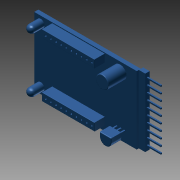
# Autodesk Inventor part: Adafruit xbee adapter
Saved by Autodesk Inventor 2012 (Build 160160000, 160)
## iProperties
Created: 2012-03-02
Part Number: Adafruit xbee adapter
Material: Default
Document SubType Name: Modeling
Designer: Lauszus
Density: 1 g/cm^3
Author: Lauszus
Autodesk Inventor part; units mm, degrees
ref_plane "YZ Plane" through (0, 0, 0) normal (1, 0, 0) x (0, 1, 0)
ref_plane "XZ Plane" through (0, 0, 0) normal (0, 1, 0) x (-1, 0, 0)
ref_plane "XY Plane" through (0, 0, 0) normal (0, 0, 1) x (1, 0, 0)
sketch "Sketch1" plane through (0, 0, 0) normal (0, 0, 1) x (1, 0, 0)
  line L0 (22.2522, -7.5943) -> (-17.7478, -7.5943)
  line L1 (-17.7478, -7.5943) -> (-17.7478, 18.9057)
  line L2 (-17.7478, 18.9057) -> (22.2522, 18.9057)
  line L3 (22.2522, 18.9057) -> (22.2522, -7.5943)
  line L4 (-10.7478, 18.5791) -> (9.7522, 18.5791)
  line L5 (9.7522, 18.5791) -> (9.7522, 15.5791)
  line L6 (9.7522, 15.5791) -> (-10.7478, 15.5791)
  line L7 (-10.7478, 15.5791) -> (-10.7478, 18.5791)
  circle A0 centre (-15.2478, -5.0275) radius 1.5
  circle A1 centre (-15.2478, 16.3389) radius 1.5
  circle A2 centre (15.7522, 15.4057) radius 2.5
  line L8 (18.2522, -4.3443) -> (18.2522, -2.8443)
  line L9 (18.2522, -2.8443) -> (13.7522, -2.8443)
  line L10 (13.7522, -2.8443) -> (13.7522, -4.3443)
  arc A3 (13.7522, -4.3443) -> (18.2522, -4.3443) centre (16.0022, -4.3443) ccw
  line L11 (14.295, -3.3443) -> (14.795, -3.3443)
  line L12 (14.795, -3.3443) -> (14.795, -3.8443)
  line L13 (14.795, -3.8443) -> (14.295, -3.8443)
  line L14 (14.295, -3.8443) -> (14.295, -3.3443)
  line L15 (15.795, -3.3443) -> (16.295, -3.3443)
  line L16 (16.295, -3.3443) -> (16.295, -3.8443)
  line L17 (16.295, -3.8443) -> (15.795, -3.8443)
  line L18 (15.795, -3.8443) -> (15.795, -3.3443)
  line L19 (17.295, -3.3443) -> (17.795, -3.3443)
  line L20 (17.795, -3.3443) -> (17.795, -3.8443)
  line L21 (17.795, -3.8443) -> (17.295, -3.8443)
  line L22 (17.295, -3.8443) -> (17.295, -3.3443)
  line L23 (-9.6556, 17.3791) -> (-9.0556, 17.3791)
  line L24 (-9.0556, 17.3791) -> (-9.0556, 16.7791)
  line L25 (-9.0556, 16.7791) -> (-9.6556, 16.7791)
  line L26 (-9.6556, 16.7791) -> (-9.6556, 17.3791)
  line L27 (-7.6556, 17.3791) -> (-7.0556, 17.3791)
  line L28 (-7.0556, 17.3791) -> (-7.0556, 16.7791)
  line L29 (-7.0556, 16.7791) -> (-7.6556, 16.7791)
  line L30 (-7.6556, 16.7791) -> (-7.6556, 17.3791)
  line L31 (-5.6556, 16.7791) -> (-5.0556, 16.7791)
  line L32 (-5.0556, 16.7791) -> (-5.0556, 17.3791)
  line L33 (-5.0556, 17.3791) -> (-5.6556, 17.3791)
  line L34 (-5.6556, 17.3791) -> (-5.6556, 16.7791)
  line L35 (-3.6556, 16.7791) -> (-3.0556, 16.7791)
  line L36 (-3.0556, 16.7791) -> (-3.0556, 17.3791)
  line L37 (-3.0556, 17.3791) -> (-3.6556, 17.3791)
  line L38 (-3.6556, 17.3791) -> (-3.6556, 16.7791)
  line L39 (-1.6556, 16.7791) -> (-1.0556, 16.7791)
  line L40 (-1.0556, 16.7791) -> (-1.0556, 17.3791)
  line L41 (-1.0556, 17.3791) -> (-1.6556, 17.3791)
  line L42 (-1.6556, 17.3791) -> (-1.6556, 16.7791)
  line L43 (0.3444, 16.7791) -> (0.9444, 16.7791)
  line L44 (0.9444, 16.7791) -> (0.9444, 17.3791)
  line L45 (0.9444, 17.3791) -> (0.3444, 17.3791)
  line L46 (0.3444, 17.3791) -> (0.3444, 16.7791)
  line L47 (2.3444, 16.7791) -> (2.9444, 16.7791)
  line L48 (2.9444, 16.7791) -> (2.9444, 17.3791)
  line L49 (2.9444, 17.3791) -> (2.3444, 17.3791)
  line L50 (2.3444, 17.3791) -> (2.3444, 16.7791)
  line L51 (4.3444, 16.7791) -> (4.9444, 16.7791)
  line L52 (4.9444, 16.7791) -> (4.9444, 17.3791)
  line L53 (4.9444, 17.3791) -> (4.3444, 17.3791)
  line L54 (4.3444, 17.3791) -> (4.3444, 16.7791)
  line L55 (6.3444, 16.7791) -> (6.9444, 16.7791)
  line L56 (6.9444, 16.7791) -> (6.9444, 17.3791)
  line L57 (6.9444, 17.3791) -> (6.3444, 17.3791)
  line L58 (6.3444, 17.3791) -> (6.3444, 16.7791)
  line L59 (8.3444, 16.7791) -> (8.9444, 16.7791)
  line L60 (8.9444, 16.7791) -> (8.9444, 17.3791)
  line L61 (8.9444, 17.3791) -> (8.3444, 17.3791)
  line L62 (8.3444, 17.3791) -> (8.3444, 16.7791)
  line L63 (-10.7478, -2.7689) -> (9.7522, -2.7689)
  line L64 (9.7522, -2.7689) -> (9.7522, -5.7689)
  line L65 (9.7522, -5.7689) -> (-10.7478, -5.7689)
  line L66 (-10.7478, -5.7689) -> (-10.7478, -2.7689)
  line L67 (-9.6556, -3.9689) -> (-9.0556, -3.9689)
  line L68 (-9.0556, -3.9689) -> (-9.0556, -4.5689)
  line L69 (-9.0556, -4.5689) -> (-9.6556, -4.5689)
  line L70 (-9.6556, -4.5689) -> (-9.6556, -3.9689)
  line L71 (-7.6556, -3.9689) -> (-7.0556, -3.9689)
  line L72 (-7.0556, -3.9689) -> (-7.0556, -4.5689)
  line L73 (-7.0556, -4.5689) -> (-7.6556, -4.5689)
  line L74 (-7.6556, -4.5689) -> (-7.6556, -3.9689)
  line L75 (-5.6556, -4.5689) -> (-5.0556, -4.5689)
  line L76 (-5.0556, -4.5689) -> (-5.0556, -3.9689)
  line L77 (-5.0556, -3.9689) -> (-5.6556, -3.9689)
  line L78 (-5.6556, -3.9689) -> (-5.6556, -4.5689)
  line L79 (-3.6556, -4.5689) -> (-3.0556, -4.5689)
  line L80 (-3.0556, -4.5689) -> (-3.0556, -3.9689)
  line L81 (-3.0556, -3.9689) -> (-3.6556, -3.9689)
  line L82 (-3.6556, -3.9689) -> (-3.6556, -4.5689)
  line L83 (-1.6556, -4.5689) -> (-1.0556, -4.5689)
  line L84 (-1.0556, -4.5689) -> (-1.0556, -3.9689)
  line L85 (-1.0556, -3.9689) -> (-1.6556, -3.9689)
  line L86 (-1.6556, -3.9689) -> (-1.6556, -4.5689)
  line L87 (0.3444, -4.5689) -> (0.9444, -4.5689)
  line L88 (0.9444, -4.5689) -> (0.9444, -3.9689)
  line L89 (0.9444, -3.9689) -> (0.3444, -3.9689)
  line L90 (0.3444, -3.9689) -> (0.3444, -4.5689)
  line L91 (2.3444, -4.5689) -> (2.9444, -4.5689)
  line L92 (2.9444, -4.5689) -> (2.9444, -3.9689)
  line L93 (2.9444, -3.9689) -> (2.3444, -3.9689)
  line L94 (2.3444, -3.9689) -> (2.3444, -4.5689)
  line L95 (4.3444, -4.5689) -> (4.9444, -4.5689)
  line L96 (4.9444, -4.5689) -> (4.9444, -3.9689)
  line L97 (4.9444, -3.9689) -> (4.3444, -3.9689)
  line L98 (4.3444, -3.9689) -> (4.3444, -4.5689)
  line L99 (6.3444, -4.5689) -> (6.9444, -4.5689)
  line L100 (6.9444, -4.5689) -> (6.9444, -3.9689)
  line L101 (6.9444, -3.9689) -> (6.3444, -3.9689)
  line L102 (6.3444, -3.9689) -> (6.3444, -4.5689)
  line L103 (8.3444, -4.5689) -> (8.9444, -4.5689)
  line L104 (8.9444, -4.5689) -> (8.9444, -3.9689)
  line L105 (8.9444, -3.9689) -> (8.3444, -3.9689)
  line L106 (8.3444, -3.9689) -> (8.3444, -4.5689)
  dimension "d0" = 40
  dimension "d1" = 26.5
  dimension "d3" = 20.5
  dimension "d4" = 3
  dimension "d6" = 7
  dimension "d8" = 3
  dimension "d9" = 3
  dimension "d10" = 1
  dimension "d11" = 1
  dimension "d12" = 5
  dimension "d13" = 4
  dimension "d14" = 1
  dimension "d23" = 1.5
  dimension "d24" = 4.5
  dimension "d28" = 1
  dimension "d29" = 4
  dimension "d33" = 0.5
  dimension "d34" = 0.5
  dimension "d35" = 0.5
  dimension "d36" = 0.5
  dimension "d37" = 0.5
  dimension "d38" = 0.5
  dimension "d39" = 1
  dimension "d40" = 1
  dimension "d41" = 0.5
  dimension "d42" = 0.5
  dimension "d43" = 0.5
  dimension "d44" = 0.4572
  dimension "d56" = 1.0668
  dimension "d58" = 1.0668
  dimension "d191" = 0.6
  dimension "d192" = 0.6
  dimension "d193" = 1.0922
  dimension "d194" = 1.2
  dimension "d195" = 0.6
  dimension "d196" = 0.6
  dimension "d197" = 2
  dimension "d198" = 1.2
  dimension "d199" = 0.6
  dimension "d200" = 0.6
  dimension "d202" = 1.2
  dimension "d203" = 0.6
  dimension "d204" = 0.6
  dimension "d205" = 2
  dimension "d206" = 2
  dimension "d207" = 2
  dimension "d208" = 0.6
  dimension "d209" = 0.6
  dimension "d210" = 1.2
  dimension "d211" = 0.6
  dimension "d212" = 0.6
  dimension "d213" = 2
  dimension "d214" = 1.2
  dimension "d215" = 0.6
  dimension "d216" = 0.6
  dimension "d217" = 2
  dimension "d218" = 1.2
  dimension "d219" = 0.6
  dimension "d220" = 0.6
  dimension "d221" = 2
  dimension "d222" = 1.2
  dimension "d223" = 0.6
  dimension "d224" = 0.6
  dimension "d225" = 2
  constraints: 214 end point, 53 parallel, 26 horizontal, 26 perpendicular, 4 centre point, 2 point on circle, 2 point on line, 2 tangent
  measures "d0" distance of L1.end L2.end
  measures "d1" distance of L0.end L1.end
  measures "d3" distance of L4.start L4.end
  measures "d4" distance of L6.end L4.start
  measures "d6" distance between parallel lines of L1 L7
  measures "d8" diameter of A1
  measures "d9" diameter of A0
  measures "d10" distance edge to line of A0 L1
  measures "d11" distance edge to line of A1 L1
  measures "d12" diameter of A2
  measures "d13" distance edge to line of A2 L3
  measures "d14" distance edge to line of A2 L2
  measures "d23" distance of L8.start L8.end
  measures "d24" distance of L8.end L9.end
  measures "d28" distance edge to line of A3 L0
  measures "d29" distance between parallel lines of L3 L8
  measures "d33" distance of L19.start L19.end
  measures "d34" distance of L19.end L20.end
  measures "d35" distance of L15.end L16.end
  measures "d36" distance of L16.end L17.end
  measures "d37" distance of L11.end L12.end
  measures "d38" distance of L12.end L13.end
  measures "d39" distance between parallel lines of L16 L22
  measures "d40" distance between parallel lines of L12 L18
  measures "d41" distance between parallel lines of L9 L19
  measures "d42" distance between parallel lines of L9 L15
  measures "d43" distance between parallel lines of L9 L11
  measures "d44" distance between parallel lines of L8 L20
  measures "d56" distance edge to line of A1 L2
  measures "d58" distance edge to line of A0 L0
  measures "d191" distance of L23.start L23.end
  measures "d192" distance of L23.end L24.end
  measures "d193" distance between parallel lines of L7 L26
  measures "d194" distance between parallel lines of L6 L25
  measures "d195" distance of L27.start L27.end
  measures "d196" distance of L27.end L28.end
  measures "d197" distance between parallel lines of L26 L30
  measures "d198" distance between parallel lines of L6 L29
  measures "d199" distance of L32.end L33.end
  measures "d200" distance of L33.end L31.start
  measures "d202" distance between parallel lines of L6 L31
  measures "d203" distance of L37.end L35.start
  measures "d204" distance of L36.end L37.end
  measures "d205" distance between parallel lines of L34 L38
  measures "d206" distance between parallel lines of L30 L34
  measures "d207" distance between parallel lines of L38 L42
  measures "d208" distance of L40.end L41.end
  measures "d209" distance of L39.end L40.end
  measures "d210" distance between parallel lines of L6 L39
  measures "d211" distance of L44.end L45.end
  measures "d212" distance of L43.end L44.end
  measures "d213" distance between parallel lines of L42 L46
  measures "d214" distance between parallel lines of L6 L43
  measures "d215" distance of L48.end L49.end
  measures "d216" distance of L47.end L48.end
  measures "d217" distance between parallel lines of L46 L50
  measures "d218" distance between parallel lines of L6 L47
  measures "d219" distance of L52.end L53.end
  measures "d220" distance of L51.end L52.end
  measures "d221" distance between parallel lines of L50 L54
  measures "d222" distance between parallel lines of L6 L51
  measures "d223" distance of L56.end L57.end
  measures "d224" distance of L55.end L56.end
  measures "d225" distance between parallel lines of L54 L58
extrude "Extrusion1" add sketch "Sketch1" against normal blind 1.6 contours L0 L1 L2 L3 | L4 L5 L6 L7 | A0 | A1 | A2 | A3 L10 L9 L8 | L11 L12 L13 L14 | L15 L16 L17 L18 | L19 L20 L21 L22 | L23 L24 L25 L26 | L27 L28 L29 L30 | L34 L33 L32 L31 | L38 L37 L36 L35 | L42 L41 L40 L39 | L46 L45 L44 L43 | L50 L49 L48 L47 | L54 L53 L52 L51 | L58 L57 L56 L55 | L62 L61 L60 L59 | L63 L64 L65 L66 | L67 L68 L69 L70 | L71 L72 L73 L74 | L78 L77 L76 L75 | L82 L81 L80 L79 | L86 L85 L84 L83 | L90 L89 L88 L87 | L94 L93 L92 L91 | L98 L97 L96 L95 | L102 L101 L100 L99 | L106 L105 L104 L103
extrude "Extrusion2" add sketch "Sketch1" along normal blind 7 contours A2
extrude "Extrusion3" add sketch "Sketch1" along normal blind 5 contours A0 | A1
fillet "Fillet1" radius 1.4986 2 edges at (-16.7478, -5.0275, 5) (-16.7478, 16.3389, 5)
fillet "Fillet2" radius 0.254 1 edges at (13.2522, 15.4057, 7)
extrude "Extrusion5" add sketch "Sketch1" along normal blind 2 contours L11 L12 L13 L14 | L15 L16 L17 L18 | L19 L20 L21 L22
sketch "Sketch3" plane through (22.2522, -7.5943, 0) normal (1, 0, 0) x (0, 0, -1)
  line L0 (0, 0) -> (1.6, 0) projected
  line L1 (0.8, 0) -> (2.5, 0)
  line L2 (2.5, 0) -> (2.5, 26.5)
  line L3 (2.5, 26.5) -> (0.8, 26.5)
  line L4 (0.8, 26.5) -> (0.8, 0)
  line L5 (1.9, 2.0621) -> (1.4, 2.0621)
  line L6 (1.4, 2.0621) -> (1.4, 1.5621)
  line L7 (1.4, 1.5621) -> (1.9, 1.5621)
  line L8 (1.9, 1.5621) -> (1.9, 2.0621)
  line L9 (1.9, 4.1021) -> (1.4, 4.1021)
  line L10 (1.4, 4.1021) -> (1.4, 4.6021)
  line L11 (1.4, 4.6021) -> (1.9, 4.6021)
  line L12 (1.9, 4.6021) -> (1.9, 4.1021)
  line L13 (1.9, 6.6421) -> (1.4, 6.6421)
  line L14 (1.4, 6.6421) -> (1.4, 7.1421)
  line L15 (1.4, 7.1421) -> (1.9, 7.1421)
  line L16 (1.9, 7.1421) -> (1.9, 6.6421)
  line L17 (1.9, 9.6821) -> (1.4, 9.6821)
  line L18 (1.4, 9.6821) -> (1.4, 9.1821)
  line L19 (1.4, 9.1821) -> (1.9, 9.1821)
  line L20 (1.9, 9.1821) -> (1.9, 9.6821)
  line L21 (1.9, 12.2221) -> (1.4, 12.2221)
  line L22 (1.4, 12.2221) -> (1.4, 11.7221)
  line L23 (1.4, 11.7221) -> (1.9, 11.7221)
  line L24 (1.9, 11.7221) -> (1.9, 12.2221)
  line L25 (1.9, 14.7621) -> (1.4, 14.7621)
  line L26 (1.4, 14.7621) -> (1.4, 14.2621)
  line L27 (1.4, 14.2621) -> (1.9, 14.2621)
  line L28 (1.9, 14.2621) -> (1.9, 14.7621)
  line L29 (1.9, 17.3021) -> (1.4, 17.3021)
  line L30 (1.4, 17.3021) -> (1.4, 16.8021)
  line L31 (1.4, 16.8021) -> (1.9, 16.8021)
  line L32 (1.9, 16.8021) -> (1.9, 17.3021)
  line L33 (1.4, 19.3421) -> (1.9, 19.3421)
  line L34 (1.9, 19.3421) -> (1.9, 19.8421)
  line L35 (1.9, 19.8421) -> (1.4, 19.8421)
  line L36 (1.4, 19.8421) -> (1.4, 19.3421)
  line L37 (1.4, 21.8821) -> (1.9, 21.8821)
  line L38 (1.9, 21.8821) -> (1.9, 22.3821)
  line L39 (1.9, 22.3821) -> (1.4, 22.3821)
  line L40 (1.4, 22.3821) -> (1.4, 21.8821)
  line L41 (1.4, 24.4221) -> (1.9, 24.4221)
  line L42 (1.9, 24.4221) -> (1.9, 24.9221)
  line L43 (1.9, 24.9221) -> (1.4, 24.9221)
  line L44 (1.4, 24.9221) -> (1.4, 24.4221)
  point P0 (0, 7.5943)
  dimension "d122" = 26.5
  dimension "d123" = 1.7
  dimension "d124" = 0.5
  dimension "d125" = 0.5
  dimension "d126" = 1.5621
  dimension "d127" = 0.6
  dimension "d128" = 0.5
  dimension "d129" = 0.5
  dimension "d130" = 0.5
  dimension "d131" = 0.5
  dimension "d145" = 0.6
  dimension "d147" = 0.6
  dimension "d148" = 0.5
  dimension "d149" = 0.5
  dimension "d150" = 2.54
  dimension "d151" = 0.6
  dimension "d152" = 2.54
  dimension "d154" = 0.5
  dimension "d155" = 0.5
  dimension "d156" = 2.54
  dimension "d157" = 0.6
  dimension "d158" = 0.5
  dimension "d159" = 0.5
  dimension "d160" = 2.54
  dimension "d161" = 0.6
  dimension "d162" = 2.54
  dimension "d163" = 0.5
  dimension "d164" = 0.5
  dimension "d166" = 2.54
  dimension "d167" = 0.6
  dimension "d168" = 0.5
  dimension "d169" = 0.5
  dimension "d170" = 2.54
  dimension "d171" = 0.6
  dimension "d172" = 0.5
  dimension "d173" = 0.5
  dimension "d174" = 2.54
  dimension "d175" = 0.6
  dimension "d176" = 0.5
  dimension "d177" = 0.5
  dimension "d178" = 2.54
  dimension "d179" = 0.6
  constraints: 88 end point, 22 parallel, 11 horizontal, 11 perpendicular, 1 midpoint
  measures "d122" distance of L1.end L2.end
  measures "d123" distance of L2.end L3.end
  measures "d124" distance of L5.end L6.end
  measures "d125" distance of L5.start L5.end
  measures "d126" distance from line of L1 L6.end
  measures "d127" distance between parallel lines of L4 L6
  measures "d128" distance of L10.end L11.end
  measures "d129" distance of L9.end L10.end
  measures "d130" distance of L15.start L15.end
  measures "d131" distance of L14.start L15.start
  measures "d145" distance between parallel lines of L4 L10
  measures "d147" distance between parallel lines of L4 L14
  measures "d148" distance of L17.end L18.end
  measures "d149" distance of L17.start L17.end
  measures "d150" distance from line of L13 L19.end
  measures "d151" distance between parallel lines of L4 L18
  measures "d152" distance between parallel lines of L7 L9
  measures "d154" distance of L21.end L22.end
  measures "d155" distance of L21.start L21.end
  measures "d156" distance between parallel lines of L19 L23
  measures "d157" distance between parallel lines of L4 L22
  measures "d158" distance of L25.end L26.end
  measures "d159" distance of L25.start L25.end
  measures "d160" distance from line of L23 L26.end
  measures "d161" distance between parallel lines of L4 L26
  measures "d162" distance between parallel lines of L9 L13
  measures "d163" distance of L29.end L30.end
  measures "d164" distance of L30.end L31.end
  measures "d166" distance between parallel lines of L27 L31
  measures "d167" distance between parallel lines of L4 L30
  measures "d168" distance of L35.end L33.start
  measures "d169" distance of L33.start L33.end
  measures "d170" distance between parallel lines of L31 L33
  measures "d171" distance between parallel lines of L4 L36
  measures "d172" distance of L39.end L37.start
  measures "d173" distance of L37.start L37.end
  measures "d174" distance between parallel lines of L33 L37
  measures "d175" distance between parallel lines of L4 L40
  measures "d176" distance of L43.end L41.start
  measures "d177" distance of L41.start L41.end
  measures "d178" distance between parallel lines of L37 L41
  measures "d179" distance between parallel lines of L4 L44
extrude "Extrusion8" add sketch "Sketch3" along normal blind 8 contours L8 L7 L6 L5 | L9 L10 L11 L12 | L13 L14 L15 L16 | L20 L19 L18 L17 | L24 L23 L22 L21 | L28 L27 L26 L25 | L32 L31 L30 L29 | L36 L35 L34 L33 | L40 L39 L38 L37 | L44 L43 L42 L41
extrude "Extrusion9" add sketch "Sketch3" along normal blind 2.5
extrude "Extrusion10" add sketch "Sketch3" against normal blind 3 contours L8 L7 L6 L5 | L9 L10 L11 L12 | L13 L14 L15 L16 | L20 L19 L18 L17 | L24 L23 L22 L21 | L28 L27 L26 L25 | L32 L31 L30 L29 | L36 L35 L34 L33 | L40 L39 L38 L37 | L44 L43 L42 L41
extrude "Extrusion11" add sketch "Sketch1" along normal blind 4 contours L4 L5 L6 L7 | L63 L64 L65 L66
fillet "Fillet6" radius 0.127 8 edges at (-0.4978, 18.5791, 4) (-10.7478, 17.0791, 4) (-0.4978, 15.5791, 4) (9.7522, 17.0791, 4) (9.7522, -4.2689, 4) (-0.4978, -2.7689, 4) (-10.7478, -4.2689, 4) (-0.4978, -5.7689, 4)
sketch "Sketch4" plane through (0, 0, 2) normal (0, 0, 1) x (1, 0, 0)
  line L0 (13.7507, -2.8338) -> (18.2451, -2.8338)
  line L1 (18.2451, -2.8338) -> (18.2451, -4.3503)
  line L2 (13.7507, -4.3503) -> (13.7507, -2.8338)
  arc A0 (13.7507, -4.3503) -> (18.2451, -4.3503) centre (15.9979, -4.3503) ccw
  point P0 (0, 0)
  constraints: 6 end point, 2 point on circle, 2 tangent, 1 centre point, 1 horizontal, 1 parallel, 1 perpendicular
extrude "Extrusion12" add sketch "Sketch4" along normal blind 4
fillet "Fillet7" radius 0.254 4 edges at (15.9979, -2.8338, 6) (13.7507, -3.5921, 6) (18.2451, -3.5921, 6) (15.9979, -6.5976, 6)
body "Solid1"
